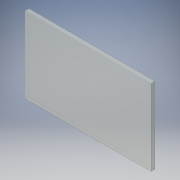
# Autodesk Inventor part: OutsideWall
Saved by Autodesk Inventor 2016 (Build 200138000, 138)
## iProperties
Created: 2016-05-26
Part Number: OutsideWall
Material: Generic
Document SubType Name: Modeling
Designer: cutrones
Density: 1 g/cm^3
Appearance: Clear
Length: 16.500 in
Height: 10.000 in
Thick: 0.500 in
Author: cutrones
Autodesk Inventor part; units mm, degrees
ref_plane "YZ Plane" through (0, 0, 0) normal (1, 0, 0) x (0, 1, 0)
ref_plane "XZ Plane" through (0, 0, 0) normal (0, 1, 0) x (-1, 0, 0)
ref_plane "XY Plane" through (0, 0, 0) normal (0, 0, 1) x (1, 0, 0)
sketch "Sketch1" plane through (0, 0, 0) normal (0, 0, 1) x (1, 0, 0)
  line L0 (0, 0) -> (419.1, 0)
  line L1 (419.1, 0) -> (419.1, 254)
  line L2 (419.1, 254) -> (0, 254)
  line L3 (0, 254) -> (0, 0)
  dimension "Length" = 419.1
  dimension "Height" = 254
  constraints: 8 end point, 2 parallel, 1 horizontal, 1 perpendicular
  measures "Length" distance of L2.end L1.end
  measures "Height" distance between parallel lines of L0 L2
extrude "Extrusion1" add sketch "Sketch1" along normal mid plane 12.7
body "Solid1"
